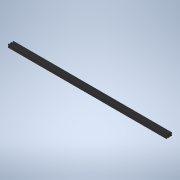
# Autodesk Inventor part: 25.02.1400(00-00-0)(0)
Saved by Autodesk Inventor 2021 (Build 250183000, 183)
## iProperties
Created: 2025-04-22
Part Number: 25.02.1400(00-00-0)(0)
Material: Generic
Catalog Web Link: www.cadenas.de
Description: Aluminium Profile mk 2025.02-Aluminium Construction Profiles Series 25
Vendor: MASCHINENBAUKITZ
Document SubType Name: Modeling
Designer: psAdmin
Manufacturer: MASCHINENBAUKITZ
Mass: 1890 g
Surface Area: 6196.21 cm^2
Volume: 702.089 cm^3
Density: 1 g/cm^3
Appearance: PSOLRGB-175-175-175
Category: PARTsolutions
Company: MASCHINENBAUKITZ
Title: 25.02.1400(00-00-0)
Author: Cadenas PARTsolutions
Comments: Aluminium Construction Profiles Series 25
L: 1400
PSOL_IDENT_0: {$CADENAS_DATA/23d-libs/maschinenbau_kitz/1_profiltechnik/1_profile/1_serie25/mk_2025_02.prj},247 {V
PSOL_IDENT_1: TYP=3D},{NB=25.02.1400(00-00-0)(0)},{LINA=25.02.1400(00-00-0)},{NN=Aluminium Profile mk 2025.02},{DA
PSOL_IDENT_2: TE=02.05.2024 06:49:00},{GEOMDATE=19.01.2024 09:41:09},{VERSION=},{LINEID=10},{WBVAR=L,MOD,ALPHA,BET
PSOL_IDENT_3: A,POS,DARST},{WBNUMERIC=L,ALPHA,BETA,DARST}  {NB=25.02.1400(00-00-0)(0)},{LINA=25.02.1400(00-00-0)},
PSOL_IDENT_4: {KT=DUMMY},{ARTIKELNR=25.02.},{L=1400},{MOD=-},{ALPHA=0},{ALPHAALG=[0:0]},{BETA=0},{BETAALG=[0:0]},{
PSOL_IDENT_5: POS=-},{DARST=0},{GW=1.35},{BZ1=Profil mk 2025.02},{MTR=AlMgSi 0,5 F25},{OBRFL=eloxiert E6/EV1},{ABM=
PSOL_IDENT_6: 25 x 50 mm},{FRB=Alu natur},{LGL=5100},{A=501.12},{IX=3.30},{IY=12.19},{WX=2.64},{WY=4.87},{O=},{GWC
PSOL_IDENT_7: ALC=1.89},{LALG=50,[1:5100]},{POSALG='-','none','../../pics/pos_none.png'},{LINAALG=25.02.1400(00-00
PSOL_IDENT_8: -0)}
NB: 25.02.1400(00-00-0)(0)
NN: Aluminium Profile mk 2025.02
NT: Aluminium Construction Profiles Series 25
NBSYN: $LINAALG.($DARST.)
LINA: 25.02.1400(00-00-0)
CATALOG: Maschinenbau Kitz
ARTIKELNR: 25.02.
MOD: none
ALPHA: 0
BETA: 0
POS: none
DARST: High
GW: 1.35
BZ1: Profile mk 2025.02
MTR: AlMgSi 0,5 F25
OBRFL: anodized E6/EV1
ABM: 25 x 50 mm
FRB: Alu natural
LGL: 5100
A: 501.12
IX: 3.3
IY: 12.19
WX: 2.64
WY: 4.87
SUPPLIER: MASCHINENBAUKITZ
ARTICLENO: 25.02.1400(00-00-0)(0)
BOMINFO: 25.02.1400(00-00-0)
CREATOR: CADENAS GmbH
Autodesk Inventor part; units mm, degrees
ref_plane "YZ Plane" through (0, 0, 0) normal (1, 0, 0) x (0, 1, 0)
ref_plane "XZ Plane" through (0, 0, 0) normal (0, 1, 0) x (-1, 0, 0)
ref_plane "XY Plane" through (0, 0, 0) normal (0, 0, 1) x (1, 0, 0)
sketch "Skizze_1" plane through (0, 0, 0) normal (1, 0, 0) x (0, 1, 0)
  line L0 (25, 0) -> (15.525, 0)
  line L1 (15.525, 0) -> (15.525, -2)
  line L2 (15.525, -2) -> (17.75, -2)
  line L3 (17.75, -2) -> (17.75, -5.5)
  line L4 (17.75, -5.5) -> (16.75, -6.5)
  line L5 (16.75, -6.5) -> (8.25, -6.5)
  line L6 (8.25, -6.5) -> (7.25, -5.5)
  line L7 (7.25, -5.5) -> (7.25, -2)
  line L8 (7.25, -2) -> (9.475, -2)
  line L9 (9.475, -2) -> (9.475, 0)
  line L10 (9.475, 0) -> (0, 0)
  line L11 (0, 0) -> (0, -9.475)
  line L12 (0, -9.475) -> (2, -9.475)
  line L13 (2, -9.475) -> (2, -7.25)
  line L14 (2, -7.25) -> (5.5, -7.25)
  line L15 (5.5, -7.25) -> (6.5, -8.25)
  line L16 (6.5, -8.25) -> (6.5, -16.75)
  line L17 (6.5, -16.75) -> (5.5, -17.75)
  line L18 (5.5, -17.75) -> (2, -17.75)
  line L19 (2, -17.75) -> (2, -15.525)
  line L20 (2, -15.525) -> (0, -15.525)
  line L21 (0, -15.525) -> (0, -34.475)
  line L22 (0, -34.475) -> (2, -34.475)
  line L23 (2, -34.475) -> (2, -32.25)
  line L24 (2, -32.25) -> (5.5, -32.25)
  line L25 (5.5, -32.25) -> (6.5, -33.25)
  line L26 (6.5, -33.25) -> (6.5, -41.75)
  line L27 (6.5, -41.75) -> (5.5, -42.75)
  line L28 (5.5, -42.75) -> (2, -42.75)
  line L29 (2, -42.75) -> (2, -40.525)
  line L30 (2, -40.525) -> (0, -40.525)
  line L31 (0, -40.525) -> (0, -50)
  line L32 (0, -50) -> (9.475, -50)
  line L33 (9.475, -50) -> (9.475, -48)
  line L34 (9.475, -48) -> (7.25, -48)
  line L35 (7.25, -48) -> (7.25, -44.5)
  line L36 (7.25, -44.5) -> (8.25, -43.5)
  line L37 (8.25, -43.5) -> (16.75, -43.5)
  line L38 (16.75, -43.5) -> (17.75, -44.5)
  line L39 (17.75, -44.5) -> (17.75, -48)
  line L40 (17.75, -48) -> (15.525, -48)
  line L41 (15.525, -48) -> (15.525, -50)
  line L42 (15.525, -50) -> (25, -50)
  line L43 (25, -50) -> (25, -40.525)
  line L44 (25, -40.525) -> (23, -40.525)
  line L45 (23, -40.525) -> (23, -42.75)
  line L46 (23, -42.75) -> (19.5, -42.75)
  line L47 (19.5, -42.75) -> (18.5, -41.75)
  line L48 (18.5, -41.75) -> (18.5, -33.25)
  line L49 (18.5, -33.25) -> (19.5, -32.25)
  line L50 (19.5, -32.25) -> (23, -32.25)
  line L51 (23, -32.25) -> (23, -34.475)
  line L52 (23, -34.475) -> (25, -34.475)
  line L53 (25, -34.475) -> (25, -15.525)
  line L54 (25, -15.525) -> (23, -15.525)
  line L55 (23, -15.525) -> (23, -17.75)
  line L56 (23, -17.75) -> (19.5, -17.75)
  line L57 (19.5, -17.75) -> (18.5, -16.75)
  line L58 (18.5, -16.75) -> (18.5, -8.25)
  line L59 (18.5, -8.25) -> (19.5, -7.25)
  line L60 (19.5, -7.25) -> (23, -7.25)
  line L61 (23, -7.25) -> (23, -9.475)
  line L62 (23, -9.475) -> (25, -9.475)
  line L63 (25, -9.475) -> (25, 0)
  circle A0 centre (3.75, -46.25) radius 2.1
  circle A1 centre (21.25, -46.25) radius 2.1
  circle A2 centre (12.5, -37.5) radius 4.25
  line L64 (8.25, -18.5) -> (6.75, -20)
  line L65 (6.75, -20) -> (3, -20)
  line L66 (3, -20) -> (2.5, -20.5)
  line L67 (2.5, -20.5) -> (2.5, -29.5)
  line L68 (2.5, -29.5) -> (3, -30)
  line L69 (3, -30) -> (6.75, -30)
  line L70 (6.75, -30) -> (8.25, -31.5)
  line L71 (8.25, -31.5) -> (16.75, -31.5)
  line L72 (16.75, -31.5) -> (18.25, -30)
  line L73 (18.25, -30) -> (22, -30)
  line L74 (22, -30) -> (22.5, -29.5)
  line L75 (22.5, -29.5) -> (22.5, -20.5)
  line L76 (22.5, -20.5) -> (22, -20)
  line L77 (22, -20) -> (18.25, -20)
  line L78 (18.25, -20) -> (16.75, -18.5)
  line L79 (16.75, -18.5) -> (8.25, -18.5)
  circle A3 centre (12.5, -12.5) radius 4.25
  circle A4 centre (3.75, -3.75) radius 2.1
  circle A5 centre (21.25, -3.75) radius 2.1
  constraints: 160 end point, 6 centre point
extrude "Extrusion1" add sketch "Skizze_1" along normal blind 1400
equation "\"d0\" = L"
equation "\"L\" = 1400"
body "Solid1"
